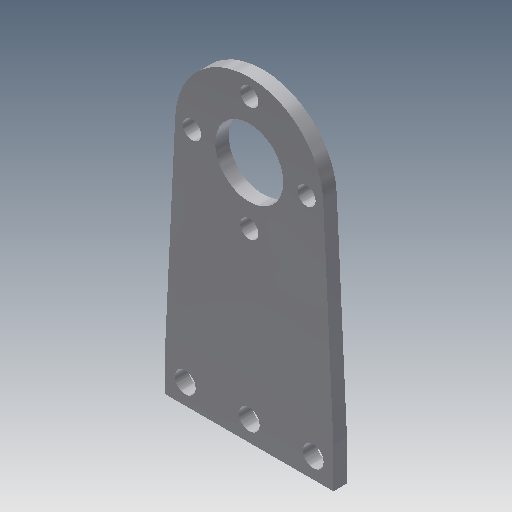
# Autodesk Inventor part: 足裏_メインフレーム_1_1
Saved by Autodesk Inventor 2017.3 (Build 213256000, 256)
## iProperties
Created: 2016-05-01
Part Number: 足裏_メインフレーム_1_1
Material: アルミニウム 2014-T4
Document SubType Name: Modeling
Designer: hiroaki
Density: 2.8 g/cm^3
Appearance: サテン
Mass: 5.15095 g
Surface Area: 22.9264 cm^2
Volume: 1.83962 cm^3
Author: hiroaki
Autodesk Inventor part; units mm, degrees
ref_plane "YZ Plane" through (0, 0, 0) normal (1, 0, 0) x (0, 1, 0)
ref_plane "XZ Plane" through (0, 0, 0) normal (0, 1, 0) x (-1, 0, 0)
ref_plane "XY Plane" through (0, 0, 0) normal (0, 0, 1) x (1, 0, 0)
derived "足裏_基礎_1.ipt"
sketch "スケッチ1" plane through (0, 0, 0) normal (0, 0, 1) x (1, 0, 0)
  circle A0 centre (0, 0) radius 5.05
  line L0 (-21.25, 26.6) -> (21.25, 26.6) construction
  line L1 (21.25, 26.6) -> (21.25, -16) construction
  line L2 (21.25, -16) -> (-21.25, -16) construction
  line L3 (-21.25, -16) -> (-21.25, 26.6) construction
  circle A1 centre (0, 0) radius 26.6 construction
  line L4 (-12.5, -36) -> (12.5, -36)
  line L5 (12.5, -36) -> (12.5, -30)
  line L6 (12.5, -30) -> (10.9865, 0.5444)
  line L7 (-12.5, -36) -> (-12.5, -30)
  line L8 (-12.5, -30) -> (-10.9865, 0.5444)
  arc A2 (10.9865, 0.5444) -> (-10.9865, 0.5444) centre (0, 0) ccw
  line L9 (12.5, -30) -> (-12.5, -30) construction
  circle A3 centre (0, 8.5) radius 1.35
  circle A4 centre (0, 8.5) radius 2.5 construction
  circle A5 centre (-8.5, 0) radius 1.35
  circle A6 centre (0, -8.5) radius 1.35
  circle A7 centre (8.5, 0) radius 1.35
  circle A8 centre (-9.5, -33) radius 1.55
  circle A9 centre (0, -33) radius 1.55
  circle A10 centre (9.5, -33) radius 1.55
  line L10 (-12.5, -33) -> (12.5, -33) construction
  line L11 (0, 0) -> (0, -30) construction
  line L12 (-6.3, -30) -> (-3.2, -30) construction
  line L13 (-3.2, -30) -> (-3.2, -36) construction
  line L14 (-3.2, -36) -> (-6.3, -36) construction
  line L15 (-6.3, -36) -> (-6.3, -30) construction
  line L16 (3.2, -30) -> (6.3, -30) construction
  line L17 (6.3, -30) -> (6.3, -36) construction
  line L18 (6.3, -36) -> (3.2, -36) construction
  line L19 (3.2, -36) -> (3.2, -30) construction
  line L20 (-4.75, -30) -> (-4.75, -36) construction
  line L21 (4.75, -30) -> (4.75, -36) construction
  point P0 (0, 26.6)
  point P1 (0, -36)
extrude "押し出し1" add sketch "スケッチ1" along normal blind 2
